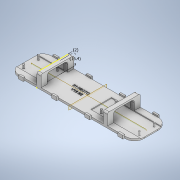
# Autodesk Inventor part: R1 Proto V13 B2
Saved by Autodesk Inventor 2021 (Build 250183000, 183)
## iProperties
Created: 2020-06-27
Part Number: R1 Proto V13 B2
Material: Generic
Document SubType Name: Modeling
Designer: andre
Density: 1 g/cm^3
Appearance: Default
Author: andre
Autodesk Inventor part; units mm, degrees
ref_plane "YZ Plane" through (0, 0, 0) normal (1, 0, 0) x (0, 1, 0)
ref_plane "XZ Plane" through (0, 0, 0) normal (0, 1, 0) x (-1, 0, 0)
ref_plane "XY Plane" through (0, 0, 0) normal (0, 0, 1) x (1, 0, 0)
sketch "Sketch1" plane through (0, 0, 0) normal (0, 1, 0) x (-1, 0, 0)
  line L0 (0, 0) -> (126, 0)
  line L1 (126, 0) -> (126, -39.4)
  line L2 (126, -39.4) -> (0, -39.4)
  line L3 (0, -39.4) -> (0, 0)
  dimension "d2" = 126
  dimension "d3" = 39.4
  constraints: 8 end point, 2 parallel, 1 horizontal, 1 perpendicular
  measures "d2" distance between parallel lines of L3 L1
  measures "d3" distance between parallel lines of L2 L0
extrude "Extrusion1" add sketch "Sketch1" along normal blind 2.4
sketch "Sketch2" plane through (-126, 0, 0) normal (0, 0, 1) x (1, 0, 0)
  line L0 (126, 0) -> (126, 2.4) projected
  line L1 (126, 0) -> (120, 0)
  line L2 (120, 0) -> (120, 2.4)
  line L3 (120, 2.4) -> (126, 2.4)
  line L4 (126, 2.4) -> (126, 0)
  line L5 (0, 0) -> (126, 0) projected
  line L6 (0, 2.4) -> (126, 2.4) projected
  line L7 (80, 2.4) -> (86, 2.4)
  line L8 (86, 2.4) -> (86, 0)
  line L9 (86, 0) -> (80, 0)
  line L10 (80, 0) -> (80, 2.4)
  point P0 (86, 0)
  dimension "d4" = 0
  dimension "d5" = 0
  dimension "d6" = 6
  dimension "d16" = 0
  dimension "d17" = 0
  dimension "d18" = 6
  dimension "d19" = 34
  constraints: 16 end point, 4 parallel, 2 horizontal, 2 perpendicular, 1 point on line
  measures "d4" distance between parallel lines of L5 L1
  measures "d5" distance between parallel lines of L6 L3
  measures "d6" distance between parallel lines of L0 L2
  measures "d16" distance between parallel lines of L6 L7
  measures "d17" distance between parallel lines of L5 L9
  measures "d18" distance between parallel lines of L8 L10
  measures "d19" distance between parallel lines of L2 L8
extrude "Extrusion2" add sketch "Sketch2" along normal blind 2 contours L1 L2 L3 L0 | L5 L10 L6 L8
sketch "Sketch3" plane through (0, 2.4, 0) normal (0, 1, 0) x (1, 0, 0)
  line L0 (-6, -2) -> (0, -2)
  line L1 (0, -2) -> (0, 0)
  line L2 (0, 0) -> (-6, 0)
  line L3 (-6, 0) -> (-6, -2)
  line L4 (-6, 0) -> (-6, -2) projected
  line L5 (0, 39.4) -> (0, -2) projected
  line L6 (0, -2) -> (-6, -2) projected
  line L7 (-126, 0) -> (-6, 0) projected
  line L8 (-46, -2) -> (-40, -2)
  line L9 (-40, -2) -> (-40, 0)
  line L10 (-40, 0) -> (-46, 0)
  line L11 (-46, 0) -> (-46, -2)
  line L12 (-46, 0) -> (-46, -2) projected
  line L13 (-40, 0) -> (-40, -2) projected
  line L14 (-40, -2) -> (-46, -2) projected
  point P0 (0, 0)
  point P1 (-40, 0)
  dimension "d9" = 0
  dimension "d10" = 0
  dimension "d11" = 0
  dimension "d12" = 0
  dimension "d20" = 0
  dimension "d21" = 0
  dimension "d22" = 0
  dimension "d23" = 0
  constraints: 16 end point, 4 parallel, 2 horizontal, 2 perpendicular
  measures "d9" distance between parallel lines of L4 L3
  measures "d10" distance between parallel lines of L5 L1
  measures "d11" distance between parallel lines of L6 L0
  measures "d12" distance between parallel lines of L7 L2
  measures "d20" distance between parallel lines of L12 L11
  measures "d21" distance between parallel lines of L13 L9
  measures "d22" distance between parallel lines of L14 L8
  measures "d23" distance between parallel lines of L7 L10
extrude "Extrusion3" add sketch "Sketch3" along normal blind 1.6
ref_plane "Work Plane1" through (0, 0, -19.7) normal (0, 0, -1) x (-1, 0, 0)
ref_plane "Work Plane2" through (-63, 0, -39.4) normal (1, 0, 0) x (0, 0, -1)
mirror "Mirror1" about plane through (0, 0, -19.7) normal (0, 0, -1) of "Extrusion2", "Extrusion3"
sketch "Sketch6" plane through (0, 0, 2) normal (1, 0, 0) x (0, 0, -1)
  line L0 (41.4, 2.4) -> (2, 2.4) projected
  line L1 (41.4, 2.4) -> (2, 2.4)
  line L2 (2, 2.4) -> (2, 0)
  line L3 (2, 0) -> (41.4, 0)
  line L4 (41.4, 0) -> (41.4, 2.4)
  constraints: 8 end point, 2 parallel, 1 horizontal, 1 perpendicular
extrude "Extrusion5" add sketch "Sketch6" along normal blind 12
fillet "Fillet2" radius 12 2 edges at (12, 1.2, 0) (12, 1.2, -39.4) curvature continuous yes
mirror "Mirror3" about plane through (-63, 0, -39.4) normal (1, 0, 0) of "Extrusion2", "Extrusion3", "Mirror1", "Fillet2", "Extrusion5"
sketch "Sketch7" plane through (0, 2.4, 0) normal (0, 1, 0) x (1, 0, 0)
  line L0 (-48, 32.2) -> (22, 32.2)
  line L1 (22, 32.2) -> (22, 7.2)
  line L2 (22, 7.2) -> (-48, 7.2)
  line L3 (-48, 7.2) -> (-48, 32.2)
  line L4 (-188, 19.7) -> (57, 19.7) projected
  line L5 (-63, 50.08) -> (-63, -10.68) projected
  line L6 (-103, 7.2) -> (-153, 7.2)
  line L7 (-153, 7.2) -> (-153, 32.2)
  line L8 (-153, 32.2) -> (-103, 32.2)
  line L9 (-103, 32.2) -> (-103, 7.2)
  point P0 (0, 0)
  dimension "d31" = 25
  dimension "d32" = 70
  dimension "d33" = 12.5
  dimension "d34" = 15
  dimension "d60" = 50
  dimension "d61" = 25
  dimension "d62" = 12.5
  dimension "d63" = 40
  constraints: 16 end point, 4 parallel, 2 horizontal, 2 perpendicular
  measures "d31" distance between parallel lines of L2 L0
  measures "d32" distance between parallel lines of L1 L3
  measures "d33" distance between parallel lines of L4 L0
  measures "d34" distance between parallel lines of L5 L3
  measures "d60" distance of L7.end L8.end
  measures "d61" distance of L6.end L7.end
  measures "d62" distance between parallel lines of L4 L6
  measures "d63" distance between parallel lines of L5 L9
extrude "Extrusion6" cut sketch "Sketch7" against normal blind 1
sketch "Sketch8" plane through (0, 1.4, 0) normal (0, 1, 0) x (1, 0, 0)
  circle A0 centre (6.973, 10.81) radius 0.9
  circle A1 centre (6.973, 28.59) radius 0.9
  circle A2 centre (-38.747, 10.81) radius 1.2
  circle A3 centre (-38.747, 28.59) radius 1.2
  line L0 (-168.0025, 19.7) -> (42.0025, 19.7) projected
  circle A4 centre (-109.5422, 10.81) radius 1.2
  circle A5 centre (-109.5422, 28.59) radius 1.2
  circle A6 centre (-132.4022, 10.81) radius 1.2
  circle A7 centre (-132.4022, 28.59) radius 1.2
  point P0 (0, 0)
  dimension "d37" = 1.8
  dimension "d38" = 1.8
  dimension "d39" = 2.4
  dimension "d40" = 2.4
  dimension "d41" = 0
  dimension "d42" = 0
  dimension "d43" = 0
  dimension "d44" = 0
  dimension "d45" = 17.78
  dimension "d46" = 45.72
  dimension "d47" = 8.89
  dimension "d64" = 2.4
  dimension "d65" = 2.4
  dimension "d66" = 2.4
  dimension "d67" = 2.4
  dimension "d68" = 0
  dimension "d69" = 0
  dimension "d70" = 0
  dimension "d71" = 0
  dimension "d72" = 22.86
  dimension "d73" = 17.78
  dimension "d74" = 8.89
  constraints: 8 centre point
  measures "d37" diameter of A0
  measures "d38" diameter of A1
  measures "d39" diameter of A3
  measures "d40" diameter of A2
  measures "d41" horizontal distance of A2.centre A3.centre
  measures "d42" vertical distance of A0.centre A2.centre
  measures "d43" horizontal distance of A1.centre A0.centre
  measures "d44" vertical distance of A3.centre A1.centre
  measures "d45" distance of A1.centre A0.centre
  measures "d46" distance of A0.centre A2.centre
  measures "d47" distance from line of L0 A3.centre
  measures "d64" diameter of A4
  measures "d65" diameter of A5
  measures "d66" diameter of A6
  measures "d67" diameter of A7
  measures "d68" vertical distance of A6.centre A4.centre
  measures "d69" vertical distance of A7.centre A5.centre
  measures "d70" horizontal distance of A7.centre A6.centre
  measures "d71" horizontal distance of A5.centre A4.centre
  measures "d72" distance of A6.centre A4.centre
  measures "d73" distance of A5.centre A4.centre
  measures "d74" distance from line of L0 A4.centre
extrude "Extrusion7" add sketch "Sketch8" along normal blind 4
sketch "Sketch13" plane through (0, 2.4, 0) normal (0, 1, 0) x (1, 0, 0)
  line L0 (-25.5, 0) -> (-20.5, 0)
  line L1 (-20.5, 0) -> (-20.5, 7.2)
  line L2 (-20.5, 7.2) -> (-25.5, 7.2)
  line L3 (-25.5, 7.2) -> (-25.5, 0)
  line L4 (-40, -2) -> (-40, 0) projected
  line L5 (-40, 0) -> (-6, 0) projected
  line L6 (11.4406, 7.2) -> (-48, 7.2) projected
  point P0 (0, 0)
  dimension "d75" = 5
  dimension "d76" = 14.5
  dimension "d77" = 0
  dimension "d78" = 0
  constraints: 8 end point, 2 parallel, 1 horizontal, 1 perpendicular
  measures "d75" distance between parallel lines of L1 L3
  measures "d76" distance between parallel lines of L3 L4
  measures "d77" distance between parallel lines of L5 L0
  measures "d78" distance between parallel lines of L6 L2
extrude "Extrusion9" add sketch "Sketch13" along normal blind 12
sketch "Sketch14" plane through (0, 14.4, 0) normal (0, 1, 0) x (1, 0, 0)
  line L0 (-25.5, 0) -> (-20.5, 0)
  line L1 (-20.5, 0) -> (-20.5, 19.7)
  line L2 (-20.5, 19.7) -> (-25.5, 19.7)
  line L3 (-25.5, 19.7) -> (-25.5, 0)
  line L4 (-25.5, 0) -> (-20.5, 0) projected
  line L5 (-168.0025, 19.7) -> (42.0025, 19.7) projected
  line L6 (-20.5, 0) -> (-20.5, 7.2) projected
  line L7 (-25.5, 7.2) -> (-25.5, 0) projected
  point P0 (0, 0)
  dimension "d81" = 0
  dimension "d82" = 0
  dimension "d83" = 0
  dimension "d84" = 0
  constraints: 8 end point, 2 parallel, 1 horizontal, 1 perpendicular
  measures "d81" distance between parallel lines of L4 L0
  measures "d82" distance between parallel lines of L5 L2
  measures "d83" distance between parallel lines of L6 L1
  measures "d84" distance between parallel lines of L7 L3
extrude "Extrusion10" add sketch "Sketch14" along normal blind 2
fillet "Fillet4" radius 2 1 edges at (-23, 16.4, 0) curvature continuous yes
mirror "Mirror4" about plane through (0, 0, -19.7) normal (0, 0, -1) of "Extrusion9", "Extrusion10", "Fillet4"
mirror "Mirror5" about plane through (-63, 0, -39.4) normal (1, 0, 0) of "Extrusion9", "Extrusion10", "Fillet4", "Mirror4"
fillet "Fillet5" radius 4 4 edges at (-103, 14.4, -7.2) (-103, 14.4, -32.2) (-23, 14.4, -32.2) (-23, 14.4, -7.2) curvature continuous yes
sketch "Sketch15" plane through (0, 2.4, 0) normal (0, 1, 0) x (1, 0, 0)
  line L0 (-87.2328, 29.7) -> (-61.8042, 29.7) construction
  line L1 (-61.8042, 29.7) -> (-61.8042, 9.7) construction
  line L2 (-61.8042, 9.7) -> (-87.2328, 9.7) construction
  line L3 (-87.2328, 9.7) -> (-87.2328, 29.7) construction
  line L4 (-168.0025, 19.7) -> (42.0025, 19.7) projected
  spline S0 degree 2 poles (-83.6719, 20.7501) (-83.527, 20.7525) (-83.3675, 20.9168) (-83.3651, 21.069) knots 0 0 0 1 2 2 2
  line L5 (-83.3651, 21.069) -> (-83.3651, 21.8612)
  line L6 (-83.3651, 21.8612) -> (-82.8458, 21.8612)
  line L7 (-82.8458, 21.8612) -> (-82.3603, 20.982)
  spline S1 degree 2 poles (-82.3603, 20.982) (-82.2903, 20.8516) (-82.155, 20.7477) (-82.0487, 20.7501) knots 0 0 0 1 2 2 2
  spline S2 degree 2 poles (-82.0487, 20.7501) (-81.9134, 20.7525) (-81.7444, 20.9071) (-81.7395, 21.0303) knots 0 0 0 1 2 2 2
  spline S3 degree 2 poles (-81.7395, 21.0303) (-81.7395, 21.081) (-81.7685, 21.1776) (-81.8047, 21.2404) knots 0 0 0 1 2 2 2
  line L8 (-81.8047, 21.2404) -> (-82.2274, 21.9699)
  spline S4 degree 2 poles (-82.2274, 21.9699) (-81.9835, 22.0762) (-81.725, 22.5062) (-81.725, 22.7839) knots 0 0 0 1 2 2 2
  spline S5 degree 2 poles (-81.725, 22.7839) (-81.7274, 23.2211) (-82.2733, 23.709) (-82.7806, 23.7139) knots 0 0 0 1 2 2 2
  line L9 (-82.7806, 23.7139) -> (-83.6719, 23.7139)
  spline S6 degree 2 poles (-83.6719, 23.7139) (-83.8168, 23.7139) (-83.9762, 23.5472) (-83.9762, 23.3975) knots 0 0 0 1 2 2 2
  line L10 (-83.9762, 23.3975) -> (-83.9762, 21.069)
  spline S7 degree 2 poles (-83.9762, 21.069) (-83.9762, 20.9168) (-83.8168, 20.7525) (-83.6719, 20.7501) knots 0 0 0 1 2 2 2
  line L11 (-83.3651, 22.3057) -> (-83.3651, 23.2356)
  line L12 (-83.3651, 23.2356) -> (-82.8458, 23.2356)
  spline S8 degree 2 poles (-82.8458, 23.2356) (-82.6163, 23.2332) (-82.3555, 22.9868) (-82.3531, 22.7719) knots 0 0 0 1 2 2 2
  spline S9 degree 2 poles (-82.3531, 22.7719) (-82.3531, 22.552) (-82.6067, 22.3081) (-82.841, 22.3057) knots 0 0 0 1 2 2 2
  line L13 (-82.841, 22.3057) -> (-83.3651, 22.3057)
  spline S10 degree 2 poles (-80.3289, 20.7501) (-80.1912, 20.7525) (-80.0294, 20.9168) (-80.027, 21.0569) knots 0 0 0 1 2 2 2
  line L14 (-80.027, 21.0569) -> (-80.027, 23.4168)
  spline S11 degree 2 poles (-80.027, 23.4168) (-80.0294, 23.5762) (-80.2105, 23.7574) (-80.3748, 23.7598) knots 0 0 0 1 2 2 2
  spline S12 degree 2 poles (-80.3748, 23.7598) (-80.4666, 23.7598) (-80.6332, 23.7139) (-80.7371, 23.6438) knots 0 0 0 1 2 2 2
  line L15 (-80.7371, 23.6438) -> (-81.3168, 23.2429)
  spline S13 degree 2 poles (-81.3168, 23.2429) (-81.3869, 23.1921) (-81.4497, 23.0834) (-81.4497, 23.0134) knots 0 0 0 1 2 2 2
  spline S14 degree 2 poles (-81.4497, 23.0134) (-81.4473, 22.9144) (-81.3289, 22.796) (-81.2347, 22.796) knots 0 0 0 1 2 2 2
  spline S15 degree 2 poles (-81.2347, 22.796) (-81.1888, 22.796) (-81.1139, 22.8202) (-81.0729, 22.8491) knots 0 0 0 1 2 2 2
  line L16 (-81.0729, 22.8491) -> (-80.6453, 23.1487)
  line L17 (-80.6453, 23.1487) -> (-80.6332, 23.1487)
  line L18 (-80.6332, 23.1487) -> (-80.6332, 21.0569)
  spline S16 degree 2 poles (-80.6332, 21.0569) (-80.6308, 20.9168) (-80.4666, 20.7525) (-80.3289, 20.7501) knots 0 0 0 1 2 2 2
  spline S17 degree 2 poles (-78.2105, 20.7549) (-78.0656, 20.7574) (-77.9062, 20.9216) (-77.9038, 21.0738) knots 0 0 0 1 2 2 2
  line L19 (-77.9038, 21.0738) -> (-77.9038, 21.7139)
  line L20 (-77.9038, 21.7139) -> (-77.3579, 21.7139)
  spline S18 degree 2 poles (-77.3579, 21.7139) (-77.0487, 21.7163) (-76.5801, 21.9651) (-76.3168, 22.4119) (-76.3168, 22.7139) knots 0 0 0 1 2 3 3 3
  spline S19 degree 2 poles (-76.3168, 22.7139) (-76.3168, 23.0158) (-76.5729, 23.4651) (-77.027, 23.7115) (-77.3289, 23.7139) knots 0 0 0 1 2 3 3 3
  line L21 (-77.3289, 23.7139) -> (-78.2105, 23.7139)
  spline S20 degree 2 poles (-78.2105, 23.7139) (-78.3555, 23.7139) (-78.5149, 23.5472) (-78.5149, 23.3975) knots 0 0 0 1 2 2 2
  line L22 (-78.5149, 23.3975) -> (-78.5149, 21.0738)
  spline S21 degree 2 poles (-78.5149, 21.0738) (-78.5149, 20.9216) (-78.3555, 20.7574) (-78.2105, 20.7549) knots 0 0 0 1 2 2 2
  line L23 (-77.9038, 22.1921) -> (-77.9038, 23.2308)
  line L24 (-77.9038, 23.2308) -> (-77.4907, 23.2308)
  spline S22 degree 2 poles (-77.4907, 23.2308) (-77.225, 23.2284) (-76.94, 22.9627) (-76.9376, 22.7115) knots 0 0 0 1 2 2 2
  spline S23 degree 2 poles (-76.9376, 22.7115) (-76.94, 22.4603) (-77.2274, 22.1946) (-77.4907, 22.1921) knots 0 0 0 1 2 2 2
  line L25 (-77.4907, 22.1921) -> (-77.9038, 22.1921)
  spline S24 degree 2 poles (-75.6502, 20.7501) (-75.5052, 20.7525) (-75.3458, 20.9168) (-75.3434, 21.069) knots 0 0 0 1 2 2 2
  line L26 (-75.3434, 21.069) -> (-75.3434, 21.8612)
  line L27 (-75.3434, 21.8612) -> (-74.8241, 21.8612)
  line L28 (-74.8241, 21.8612) -> (-74.3386, 20.982)
  spline S25 degree 2 poles (-74.3386, 20.982) (-74.2685, 20.8516) (-74.1332, 20.7477) (-74.027, 20.7501) knots 0 0 0 1 2 2 2
  spline S26 degree 2 poles (-74.027, 20.7501) (-73.8917, 20.7525) (-73.7226, 20.9071) (-73.7178, 21.0303) knots 0 0 0 1 2 2 2
  spline S27 degree 2 poles (-73.7178, 21.0303) (-73.7178, 21.081) (-73.7468, 21.1776) (-73.783, 21.2404) knots 0 0 0 1 2 2 2
  line L29 (-73.783, 21.2404) -> (-74.2057, 21.9699)
  spline S28 degree 2 poles (-74.2057, 21.9699) (-73.9617, 22.0762) (-73.7033, 22.5062) (-73.7033, 22.7839) knots 0 0 0 1 2 2 2
  spline S29 degree 2 poles (-73.7033, 22.7839) (-73.7057, 23.2211) (-74.2516, 23.709) (-74.7589, 23.7139) knots 0 0 0 1 2 2 2
  line L30 (-74.7589, 23.7139) -> (-75.6502, 23.7139)
  spline S30 degree 2 poles (-75.6502, 23.7139) (-75.7951, 23.7139) (-75.9545, 23.5472) (-75.9545, 23.3975) knots 0 0 0 1 2 2 2
  line L31 (-75.9545, 23.3975) -> (-75.9545, 21.069)
  spline S31 degree 2 poles (-75.9545, 21.069) (-75.9545, 20.9168) (-75.7951, 20.7525) (-75.6502, 20.7501) knots 0 0 0 1 2 2 2
  line L32 (-75.3434, 22.3057) -> (-75.3434, 23.2356)
  line L33 (-75.3434, 23.2356) -> (-74.8241, 23.2356)
  spline S32 degree 2 poles (-74.8241, 23.2356) (-74.5946, 23.2332) (-74.3337, 22.9868) (-74.3313, 22.7719) knots 0 0 0 1 2 2 2
  spline S33 degree 2 poles (-74.3313, 22.7719) (-74.3313, 22.552) (-74.5849, 22.3081) (-74.8192, 22.3057) knots 0 0 0 1 2 2 2
  line L34 (-74.8192, 22.3057) -> (-75.3434, 22.3057)
  spline S34 degree 2 poles (-71.9859, 20.7453) (-71.5511, 20.7477) (-70.9207, 21.1124) (-70.5801, 21.7863) (-70.5777, 22.2525) knots 0 0 0 1 2 3 3 3
  spline S35 degree 2 poles (-70.5777, 22.2525) (-70.5801, 22.7211) (-70.9207, 23.3975) (-71.5511, 23.7622) (-71.9859, 23.7646) knots 0 0 0 1 2 3 3 3
  spline S36 degree 2 poles (-71.9859, 23.7646) (-72.4207, 23.7622) (-73.0511, 23.3975) (-73.3917, 22.7211) (-73.3941, 22.2525) knots 0 0 0 1 2 3 3 3
  spline S37 degree 2 poles (-73.3941, 22.2525) (-73.3917, 21.7863) (-73.0511, 21.1124) (-72.4207, 20.7477) (-71.9859, 20.7453) knots 0 0 0 1 2 3 3 3
  spline S38 degree 2 poles (-71.9859, 21.2549) (-72.3506, 21.2598) (-72.7661, 21.7888) (-72.7709, 22.2525) knots 0 0 0 1 2 2 2
  spline S39 degree 2 poles (-72.7709, 22.2525) (-72.7661, 22.7187) (-72.3482, 23.2501) (-71.9859, 23.2549) knots 0 0 0 1 2 2 2
  spline S40 degree 2 poles (-71.9859, 23.2549) (-71.6236, 23.2501) (-71.2057, 22.7187) (-71.2033, 22.2525) knots 0 0 0 1 2 2 2
  spline S41 degree 2 poles (-71.2033, 22.2525) (-71.2057, 21.7888) (-71.6236, 21.2598) (-71.9859, 21.2549) knots 0 0 0 1 2 2 2
  spline S42 degree 2 poles (-69.1816, 20.7549) (-69.0366, 20.7574) (-68.8772, 20.9216) (-68.8748, 21.0738) knots 0 0 0 1 2 2 2
  line L35 (-68.8748, 21.0738) -> (-68.8748, 23.209)
  line L36 (-68.8748, 23.209) -> (-68.2709, 23.209)
  spline S43 degree 2 poles (-68.2709, 23.209) (-68.1453, 23.209) (-67.998, 23.3419) (-67.9956, 23.4603) knots 0 0 0 1 2 2 2
  spline S44 degree 2 poles (-67.9956, 23.4603) (-67.9956, 23.581) (-68.1453, 23.7139) (-68.2709, 23.7139) knots 0 0 0 1 2 2 2
  line L37 (-68.2709, 23.7139) -> (-70.0898, 23.7139)
  spline S45 degree 2 poles (-70.0898, 23.7139) (-70.2178, 23.7139) (-70.3651, 23.581) (-70.3675, 23.4603) knots 0 0 0 1 2 2 2
  spline S46 degree 2 poles (-70.3675, 23.4603) (-70.3651, 23.3419) (-70.2154, 23.209) (-70.0898, 23.209) knots 0 0 0 1 2 2 2
  line L38 (-70.0898, 23.209) -> (-69.4859, 23.209)
  line L39 (-69.4859, 23.209) -> (-69.4859, 21.0738)
  spline S47 degree 2 poles (-69.4859, 21.0738) (-69.4859, 20.9216) (-69.3265, 20.7574) (-69.1816, 20.7549) knots 0 0 0 1 2 2 2
  spline S48 degree 2 poles (-66.3748, 20.7453) (-65.94, 20.7477) (-65.3096, 21.1124) (-64.969, 21.7863) (-64.9666, 22.2525) knots 0 0 0 1 2 3 3 3
  spline S49 degree 2 poles (-64.9666, 22.2525) (-64.969, 22.7211) (-65.3096, 23.3975) (-65.94, 23.7622) (-66.3748, 23.7646) knots 0 0 0 1 2 3 3 3
  spline S50 degree 2 poles (-66.3748, 23.7646) (-66.8096, 23.7622) (-67.44, 23.3975) (-67.7806, 22.7211) (-67.783, 22.2525) knots 0 0 0 1 2 3 3 3
  spline S51 degree 2 poles (-67.783, 22.2525) (-67.7806, 21.7863) (-67.44, 21.1124) (-66.8096, 20.7477) (-66.3748, 20.7453) knots 0 0 0 1 2 3 3 3
  spline S52 degree 2 poles (-66.3748, 21.2549) (-66.7395, 21.2598) (-67.155, 21.7888) (-67.1598, 22.2525) knots 0 0 0 1 2 2 2
  spline S53 degree 2 poles (-67.1598, 22.2525) (-67.155, 22.7187) (-66.7371, 23.2501) (-66.3748, 23.2549) knots 0 0 0 1 2 2 2
  spline S54 degree 2 poles (-66.3748, 23.2549) (-66.0125, 23.2501) (-65.5946, 22.7187) (-65.5922, 22.2525) knots 0 0 0 1 2 2 2
  spline S55 degree 2 poles (-65.5922, 22.2525) (-65.5946, 21.7888) (-66.0125, 21.2598) (-66.3748, 21.2549) knots 0 0 0 1 2 2 2
  spline S56 degree 2 poles (-79.8047, 15.6596) (-79.6284, 15.6596) (-79.4038, 15.8286) (-79.3386, 16.0122) knots 0 0 0 1 2 2 2
  line L40 (-79.3386, 16.0122) -> (-78.5197, 18.2151)
  spline S57 degree 2 poles (-78.5197, 18.2151) (-78.4907, 18.2972) (-78.4907, 18.3769) knots 0 0 0 1 1 1
  spline S58 degree 2 poles (-78.4907, 18.3769) (-78.4931, 18.505) (-78.6622, 18.6571) (-78.8047, 18.6596) knots 0 0 0 1 2 2 2
  spline S59 degree 2 poles (-78.8047, 18.6596) (-78.9231, 18.6596) (-79.068, 18.546) (-79.1067, 18.4253) knots 0 0 0 1 2 2 2
  line L41 (-79.1067, 18.4253) -> (-79.7878, 16.3286)
  line L42 (-79.7878, 16.3286) -> (-79.8023, 16.3286)
  line L43 (-79.8023, 16.3286) -> (-80.4859, 18.418)
  spline S60 degree 2 poles (-80.4859, 18.418) (-80.5221, 18.5436) (-80.6743, 18.6596) (-80.7975, 18.6596) knots 0 0 0 1 2 2 2
  spline S61 degree 2 poles (-80.7975, 18.6596) (-80.9448, 18.6571) (-81.1163, 18.5001) (-81.1188, 18.3697) knots 0 0 0 1 2 2 2
  spline S62 degree 2 poles (-81.1188, 18.3697) (-81.1188, 18.2827) (-81.0898, 18.1982) knots 0 0 0 1 1 1
  line L44 (-81.0898, 18.1982) -> (-80.2758, 16.0146)
  spline S63 degree 2 poles (-80.2758, 16.0146) (-80.2105, 15.8286) (-79.9835, 15.6596) (-79.8047, 15.6596) knots 0 0 0 1 2 2 2
  spline S64 degree 2 poles (-77.1598, 15.6547) (-77.0221, 15.6571) (-76.8603, 15.8214) (-76.8579, 15.9615) knots 0 0 0 1 2 2 2
  line L45 (-76.8579, 15.9615) -> (-76.8579, 18.3214)
  spline S65 degree 2 poles (-76.8579, 18.3214) (-76.8603, 18.4808) (-77.0415, 18.662) (-77.2057, 18.6644) knots 0 0 0 1 2 2 2
  spline S66 degree 2 poles (-77.2057, 18.6644) (-77.2975, 18.6644) (-77.4642, 18.6185) (-77.568, 18.5484) knots 0 0 0 1 2 2 2
  line L46 (-77.568, 18.5484) -> (-78.1477, 18.1475)
  spline S67 degree 2 poles (-78.1477, 18.1475) (-78.2178, 18.0967) (-78.2806, 17.9881) (-78.2806, 17.918) knots 0 0 0 1 2 2 2
  spline S68 degree 2 poles (-78.2806, 17.918) (-78.2782, 17.819) (-78.1598, 17.7006) (-78.0656, 17.7006) knots 0 0 0 1 2 2 2
  spline S69 degree 2 poles (-78.0656, 17.7006) (-78.0197, 17.7006) (-77.9448, 17.7248) (-77.9038, 17.7538) knots 0 0 0 1 2 2 2
  line L47 (-77.9038, 17.7538) -> (-77.4762, 18.0533)
  line L48 (-77.4762, 18.0533) -> (-77.4642, 18.0533)
  line L49 (-77.4642, 18.0533) -> (-77.4642, 15.9615)
  spline S70 degree 2 poles (-77.4642, 15.9615) (-77.4617, 15.8214) (-77.2975, 15.6571) (-77.1598, 15.6547) knots 0 0 0 1 2 2 2
  spline S71 degree 2 poles (-75.1163, 15.633) (-74.7758, 15.6354) (-74.2661, 15.8528) (-73.9811, 16.2489) (-73.9787, 16.517) knots 0 0 0 1 2 3 3 3
  spline S72 degree 2 poles (-73.9787, 16.517) (-73.9835, 16.819) (-74.3651, 17.1813) (-74.696, 17.2151) knots 0 0 0 1 2 2 2
  line L50 (-74.696, 17.2151) -> (-74.696, 17.2272)
  spline S73 degree 2 poles (-74.696, 17.2272) (-74.4328, 17.2803) (-74.0922, 17.6306) (-74.0874, 17.9108) knots 0 0 0 1 2 2 2
  spline S74 degree 2 poles (-74.0874, 17.9108) (-74.0898, 18.1451) (-74.3458, 18.4929) (-74.8096, 18.6813) (-75.1212, 18.6837) knots 0 0 0 1 2 3 3 3
  spline S75 degree 2 poles (-75.1212, 18.6837) (-75.5101, 18.6789) (-76.0004, 18.3794) (-76.0994, 18.1596) knots 0 0 0 1 2 2 2
  spline S76 degree 2 poles (-76.0994, 18.1596) (-76.1212, 18.1088) (-76.1429, 18.0146) (-76.1429, 17.9639) knots 0 0 0 1 2 2 2
  spline S77 degree 2 poles (-76.1429, 17.9639) (-76.1429, 17.8504) (-76.0149, 17.7175) (-75.8869, 17.7151) knots 0 0 0 1 2 2 2
  spline S78 degree 2 poles (-75.8869, 17.7151) (-75.7854, 17.7151) (-75.6598, 17.8021) (-75.6115, 17.9035) knots 0 0 0 1 2 2 2
  spline S79 degree 2 poles (-75.6115, 17.9035) (-75.5415, 18.0581) (-75.3023, 18.2151) (-75.1188, 18.2151) knots 0 0 0 1 2 2 2
  spline S80 degree 2 poles (-75.1188, 18.2151) (-74.8965, 18.2127) (-74.6671, 18.0025) (-74.6671, 17.8238) knots 0 0 0 1 2 2 2
  spline S81 degree 2 poles (-74.6671, 17.8238) (-74.6695, 17.6426) (-74.9376, 17.4204) (-75.1695, 17.418) knots 0 0 0 1 2 2 2
  line L51 (-75.1695, 17.418) -> (-75.2903, 17.418)
  spline S82 degree 2 poles (-75.2903, 17.418) (-75.4014, 17.418) (-75.5221, 17.2996) (-75.5221, 17.203) knots 0 0 0 1 2 2 2
  spline S83 degree 2 poles (-75.5221, 17.203) (-75.5221, 17.1016) (-75.4014, 16.9856) (-75.2903, 16.9832) knots 0 0 0 1 2 2 2
  line L52 (-75.2903, 16.9832) -> (-75.1622, 16.9832)
  spline S84 degree 2 poles (-75.1622, 16.9832) (-74.8941, 16.9832) (-74.6018, 16.7562) (-74.6018, 16.5412) knots 0 0 0 1 2 2 2
  spline S85 degree 2 poles (-74.6018, 16.5412) (-74.6043, 16.3576) (-74.8796, 16.1281) (-75.1067, 16.1257) knots 0 0 0 1 2 2 2
  spline S86 degree 2 poles (-75.1067, 16.1257) (-75.3313, 16.1257) (-75.597, 16.2972) (-75.6719, 16.4518) knots 0 0 0 1 2 2 2
  spline S87 degree 2 poles (-75.6719, 16.4518) (-75.7154, 16.5339) (-75.841, 16.6112) (-75.9303, 16.6112) knots 0 0 0 1 2 2 2
  spline S88 degree 2 poles (-75.9303, 16.6112) (-76.0584, 16.6088) (-76.1985, 16.4736) (-76.2009, 16.3552) knots 0 0 0 1 2 2 2
  spline S89 degree 2 poles (-76.2009, 16.3552) (-76.2009, 16.3093) (-76.1767, 16.2127) (-76.1526, 16.162) knots 0 0 0 1 2 2 2
  spline S90 degree 2 poles (-76.1526, 16.162) (-76.0849, 16.017) (-75.8096, 15.7779) (-75.3965, 15.6354) (-75.1163, 15.633) knots 0 0 0 1 2 3 3 3
  line L53 (-72.4303, 15.6982) -> (-71.4424, 15.6982)
  spline S91 degree 2 poles (-71.4424, 15.6982) (-70.969, 15.703) (-70.4376, 16.1451) (-70.4328, 16.5339) knots 0 0 0 1 2 2 2
  spline S92 degree 2 poles (-70.4328, 16.5339) (-70.4376, 16.8286) (-70.8168, 17.2127) (-71.1212, 17.2417) knots 0 0 0 1 2 2 2
  line L54 (-71.1212, 17.2417) -> (-71.1212, 17.2562)
  spline S93 degree 2 poles (-71.1212, 17.2562) (-70.882, 17.2972) (-70.5777, 17.6451) (-70.5729, 17.8914) knots 0 0 0 1 2 2 2
  spline S94 degree 2 poles (-70.5729, 17.8914) (-70.5753, 18.2296) (-71.0487, 18.6161) (-71.4642, 18.6185) knots 0 0 0 1 2 2 2
  line L55 (-71.4642, 18.6185) -> (-72.4303, 18.6185)
  spline S95 degree 2 poles (-72.4303, 18.6185) (-72.5753, 18.6185) (-72.7347, 18.4518) (-72.7347, 18.3021) knots 0 0 0 1 2 2 2
  line L56 (-72.7347, 18.3021) -> (-72.7347, 16.017)
  spline S96 degree 2 poles (-72.7347, 16.017) (-72.7347, 15.8649) (-72.5753, 15.6982) (-72.4303, 15.6982) knots 0 0 0 1 2 2 2
  line L57 (-72.1236, 16.1547) -> (-72.1236, 17.0025)
  line L58 (-72.1236, 17.0025) -> (-71.6115, 17.0025)
  spline S97 degree 2 poles (-71.6115, 17.0025) (-71.341, 17.0001) (-71.056, 16.7876) (-71.056, 16.5823) knots 0 0 0 1 2 2 2
  spline S98 degree 2 poles (-71.056, 16.5823) (-71.056, 16.3721) (-71.3337, 16.1547) (-71.5994, 16.1547) knots 0 0 0 1 2 2 2
  line L59 (-71.5994, 16.1547) -> (-72.1236, 16.1547)
  line L60 (-72.1236, 17.4035) -> (-72.1236, 18.1644)
  line L61 (-72.1236, 18.1644) -> (-71.6236, 18.1644)
  spline S99 degree 2 poles (-71.6236, 18.1644) (-71.4062, 18.162) (-71.1743, 17.9711) (-71.1743, 17.7948) knots 0 0 0 1 2 2 2
  spline S100 degree 2 poles (-71.1743, 17.7948) (-71.1743, 17.6088) (-71.44, 17.4059) (-71.6864, 17.4035) knots 0 0 0 1 2 2 2
  line L62 (-71.6864, 17.4035) -> (-72.1236, 17.4035)
  line L63 (-69.8361, 15.6982) -> (-68.2202, 15.6982)
  spline S101 degree 2 poles (-68.2202, 15.6982) (-68.0994, 15.7006) (-67.9666, 15.831) (-67.9666, 15.9422) knots 0 0 0 1 2 2 2
  spline S102 degree 2 poles (-67.9666, 15.9422) (-67.9666, 16.0533) (-68.0994, 16.1837) (-68.2202, 16.1837) knots 0 0 0 1 2 2 2
  line L64 (-68.2202, 16.1837) -> (-69.3217, 16.1837)
  line L65 (-69.3217, 16.1837) -> (-69.3217, 16.1958)
  line L66 (-69.3217, 16.1958) -> (-68.6888, 16.8045)
  spline S103 degree 2 poles (-68.6888, 16.8045) (-68.4521, 17.0267) (-68.1646, 17.3576) (-68.0366, 17.6596) (-68.0366, 17.8335) knots 0 0 0 1 2 3 3 3
  spline S104 degree 2 poles (-68.0366, 17.8335) (-68.039, 18.0871) (-68.2975, 18.4687) (-68.7613, 18.6813) (-69.0729, 18.6837) knots 0 0 0 1 2 3 3 3
  spline S105 degree 2 poles (-69.0729, 18.6837) (-69.3506, 18.6813) (-69.7709, 18.505) (-70.0415, 18.2224) (-70.0922, 18.0581) knots 0 0 0 1 2 3 3 3
  spline S106 degree 2 poles (-70.0922, 18.0581) (-70.1018, 18.0267) (-70.1139, 17.9615) (-70.1139, 17.9277) knots 0 0 0 1 2 2 2
  spline S107 degree 2 poles (-70.1139, 17.9277) (-70.1139, 17.8117) (-69.9762, 17.6789) (-69.8531, 17.6789) knots 0 0 0 1 2 2 2
  spline S108 degree 2 poles (-69.8531, 17.6789) (-69.7564, 17.6765) (-69.6308, 17.7658) (-69.5825, 17.8552) knots 0 0 0 1 2 2 2
  spline S109 degree 2 poles (-69.5825, 17.8552) (-69.5028, 18.0315) (-69.2564, 18.2079) (-69.0801, 18.2079) knots 0 0 0 1 2 2 2
  spline S110 degree 2 poles (-69.0801, 18.2079) (-68.8796, 18.2054) (-68.6357, 17.9784) (-68.6332, 17.7948) knots 0 0 0 1 2 2 2
  spline S111 degree 2 poles (-68.6332, 17.7948) (-68.6308, 17.6934) (-68.7081, 17.5025) (-68.9062, 17.2682) (-69.0849, 17.0967) knots 0 0 0 1 2 3 3 3
  line L67 (-69.0849, 17.0967) -> (-69.9569, 16.2658)
  spline S112 degree 2 poles (-69.9569, 16.2658) (-70.0487, 16.1813) (-70.126, 16.0436) (-70.1236, 15.9591) knots 0 0 0 1 2 2 2
  spline S113 degree 2 poles (-70.1236, 15.9591) (-70.1236, 15.8431) (-69.9811, 15.7006) (-69.8361, 15.6982) knots 0 0 0 1 2 2 2
  point P0 (0, 0)
  dimension "d90" = 20
  dimension "d91" = 10
  constraints: 2 other
  measures "d90" distance between parallel lines of L2 L0
  measures "d91" distance between parallel lines of L4 L2
extrude "Extrusion11" cut sketch "Sketch15" against normal blind 1
sketch "Sketch16" plane through (-105.5, 2.4, -39.4) normal (-1, 0, 0) x (0, 0, 1)
  line L0 (27.4, -2.4) -> (12, -2.4) projected
  line L1 (2, 14) -> (37.4, 14) projected
  line L2 (28.2, 12) -> (11.2, 12) projected
  point P0 (39.4, -2.4)
  dimension "d94" = 16.4
  dimension "d95" = 2
  measures "d94" distance between parallel lines of L0 L1
  measures "d95" distance between parallel lines of L2 L1
equation "\"d18\" = d6"
equation "\"d30\" = d28"
equation "\"d33\" = 0.5 * d31"
equation "\"d62\" = 0.5 * d61"
equation "\"d38\" = d37"
equation "\"d39\" = d40"
equation "\"d47\" = 0.5 * d45"
equation "\"d65\" = d64"
equation "\"d66\" = d64"
equation "\"d67\" = d64"
equation "\"d74\" = 0.5 * d73"
equation "\"d76\" = 0.5 * d19 - 0.5 * d75"
equation "\"d91\" = 0.5 * d90"
equation "\"d28\" = 12"
body "Solid1"
